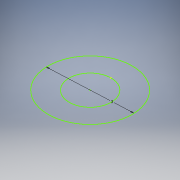
# Autodesk Inventor part: paddle
Saved by Autodesk Inventor 2018 (Build 220112000, 112)
## iProperties
Created: 2017-11-12
Part Number: paddle
Material: Generic
Document SubType Name: Sheet Metal
Designer: leo2a
Density: 1 g/cm^3
Sheet Metal Rule: Default
Appearance: Default
Author: leo2a
Autodesk Inventor part; units mm, degrees
ref_plane "YZ Plane" through (0, 0, 0) normal (1, 0, 0) x (0, 1, 0)
ref_plane "XZ Plane" through (0, 0, 0) normal (0, 1, 0) x (-1, 0, 0)
ref_plane "XY Plane" through (0, 0, 0) normal (0, 0, 1) x (1, 0, 0)
sketch "Sketch1" plane through (0, 0, 0) normal (0, 0, 1) x (1, 0, 0)
  circle A0 centre (0, -0.75) radius 0.75
  circle A1 centre (0, -0.75) radius 1.5
  line L0 (1.5, -0.75) -> (1.5, 2.25)
  line L1 (-1.5, -0.75) -> (-1.5, 2.25)
  line L2 (-1.5, 2.25) -> (1.5, 2.25)
  point P0 (0, 0)
  dimension "d1" = 3
  dimension "d2" = 3
  measures "d1" diameter of A1
  measures "d2" distance of L0.start L0.end
sketch "Sketch2" plane through (-1.5, 2.25, 0) normal (0, 1, 0) x (1, 0, 0)
  line L0 (3, 0) -> (3, 0.25)
  line L1 (3, 0.25) -> (18, 0.25)
  line L2 (18, 0.25) -> (18, 4.75)
  line L3 (18, 4.75) -> (3, 4.75)
  line L4 (3, 4.75) -> (3, 5)
  line L5 (0, 0) -> (0, 5)
  line L6 (0, 5) -> (3, 5)
  line L7 (3, 0) -> (0, 0)
  point P0 (1.5, 0)
  dimension "d4" = 0.25
  dimension "d5" = 15
  dimension "d6" = 4.5
  dimension "d7" = 0.25
  measures "d4" distance of L0.start L0.end
  measures "d5" distance of L0.end L1.end
  measures "d6" distance of L1.end L2.end
  measures "d7" distance of L3.end L4.end
extrude "Plate1" add sketch "Sketch1" along normal blind 0.5
sheet face with bend "Face2" sketch "Sketch2" thickness 0.5 toward (0, -1, 0) bend radius 0.1 relief tear relief width 0.5 relief depth 0.25
bend "Bend1"
equation "\"d3\" = Thickness"
equation "\"d9\" = BendReliefWidth"
equation "\"d11\" = MinimumRemnant"
equation "\"d10\" = BendReliefDepth"
equation "\"d12\" = TransitionRadius"
equation "\"BendRadius\" = Thickness"
equation "\"BendReliefWidth\" = Thickness"
equation "\"BendReliefDepth\" = 0.5 * Thickness"
equation "\"CornerReliefSize\" = 4 * Thickness"
equation "\"MinimumRemnant\" = 2 * Thickness"
equation "\"TransitionRadius\" = BendRadius"
equation "\"JacobiRadiusSize\" = Thickness"
equation "\"GapSize\" = Thickness"
equation "\"Thickness\" = 0.5"
body "Solid1"
